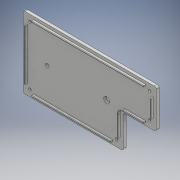
# Autodesk Inventor part: LID Enclosure Box
Saved by Autodesk Inventor 2017 (Build 210142000, 142)
## iProperties
Created: 2019-08-08
Part Number: LID Enclosure Box
Material: Generic
Document SubType Name: Modeling
Designer: harneet
Density: 1 g/cm^3
Appearance: Default
Author: harneet
Autodesk Inventor part; units mm, degrees
ref_plane "YZ Plane" through (0, 0, 0) normal (1, 0, 0) x (0, 1, 0)
ref_plane "XZ Plane" through (0, 0, 0) normal (0, 1, 0) x (-1, 0, 0)
ref_plane "XY Plane" through (0, 0, 0) normal (0, 0, 1) x (1, 0, 0)
sketch "Sketch1" plane through (0, 0, 0) normal (0, 1, 0) x (-1, 0, 0)
  line L0 (70.5, -36) -> (70.5, 36)
  line L1 (70.5, -38) -> (142.5, -38) construction
  line L2 (68.5, 38) -> (-68.5, 38)
  line L3 (-70.5, 36) -> (-70.5, -1)
  line L4 (-68.5, -3) -> (-37.5, -3)
  line L5 (68.5, -38) -> (-33.5, -38)
  line L6 (-35.5, -36) -> (-35.5, -5)
  arc A0 (70.5, 36) -> (68.5, 38) centre (68.5, 36) ccw
  arc A1 (68.5, -38) -> (70.5, -36) centre (68.5, -36) ccw
  arc A2 (-35.5, -36) -> (-33.5, -38) centre (-33.5, -36) ccw
  arc A3 (-35.5, -5) -> (-37.5, -3) centre (-37.5, -5) ccw
  arc A4 (-70.5, -1) -> (-68.5, -3) centre (-68.5, -1) ccw
  arc A5 (-68.5, 38) -> (-70.5, 36) centre (-68.5, 36) ccw
  point P0 (0, 0)
  point P1 (70.5, 38)
  point P2 (-70.5, 38)
  point P3 (-70.5, -3)
  point P4 (-35.5, -3)
  point P5 (-35.5, -38)
  dimension "d0" = 76
  dimension "d1" = 90
  dimension "d2" = 141
  dimension "d3" = 90
  dimension "d4" = 41
  dimension "d5" = 35
  dimension "d6" = 106
  dimension "d7" = 38
  dimension "d8" = 70.5
  dimension "d9" = 2
  constraints: 14 end point, 12 point on circle, 12 point on line, 12 tangent, 6 centre point, 5 equal radius, 4 perpendicular, 1 horizontal, 1 parallel, 1 vertical
  measures "d0" distance of L1.start point (70.5, 38)
  measures "d1" angle of L1 L0
  measures "d2" distance of point (70.5, 38) point (-70.5, 38)
  measures "d3" angle of L2 L0
  measures "d4" distance of point (-70.5, 38) point (-70.5, -3)
  measures "d5" distance of point (-70.5, -3) point (-35.5, -3)
  measures "d6" distance of L1.start point (-35.5, -38)
  measures "d7" distance from line of L5 point (0, 0)
  measures "d8" distance from line of L0 point (0, 0)
  measures "d9" radius of A0
extrude "Extrusion1" add sketch "Sketch1" along normal blind 3
sketch "Sketch2" plane through (0, 3, 0) normal (0, 1, 0) x (1, 0, 0)
  line L0 (-70.5, 36) -> (-70.5, -36) projected
  arc A0 (-70.5, -36) -> (-68.5, -38) centre (-68.5, -36) ccw projected
  line L1 (-68.5, -38) -> (68.5, -38) projected
  arc A1 (68.5, -38) -> (70.5, -36) centre (68.5, -36) ccw projected
  line L2 (70.5, -36) -> (70.5, 1) projected
  arc A2 (70.5, 1) -> (68.5, 3) centre (68.5, 1) ccw projected
  line L3 (68.5, 3) -> (37.5, 3) projected
  arc A3 (35.5, 5) -> (37.5, 3) centre (37.5, 5) ccw projected
  line L4 (35.5, 5) -> (35.5, 36) projected
  arc A4 (35.5, 36) -> (33.5, 38) centre (33.5, 36) ccw projected
  line L5 (33.5, 38) -> (-68.5, 38) projected
  arc A5 (-68.5, 38) -> (-70.5, 36) centre (-68.5, 36) ccw projected
  line L6 (-67.4, -27) -> (-67.4, 27)
  line L7 (-59.5, 34.9) -> (24.5, 34.9)
  line L8 (32.4, 27) -> (32.4, 5)
  arc A6 (32.4, 5) -> (37.5, -0.1) centre (37.5, 5) ccw
  line L9 (37.5, -0.1) -> (59.5, -0.1)
  line L10 (59.5, -34.9) -> (-59.5, -34.9)
  line L11 (0, 53.7799) -> (0, -53.7799) projected
  line L12 (99.2799, 0) -> (-99.2799, 0) projected
  line L13 (59.5, -33.5) -> (-59.5, -33.5)
  line L14 (-66, -27) -> (-66, 27)
  line L15 (-59.5, 33.5) -> (24.5, 33.5)
  line L16 (31, 27) -> (31, 5)
  arc A7 (31, 5) -> (37.5, -1.5) centre (37.5, 5) ccw
  line L17 (37.5, -1.5) -> (59.5, -1.5)
  line L18 (66, -8) -> (66, -27)
  line L19 (67.4, -8) -> (67.4, -27)
  line L20 (24.5, 34.9) -> (24.5, 33.5)
  line L21 (31, 27) -> (32.4, 27)
  line L22 (59.5, -1.5) -> (59.5, -0.1)
  line L23 (66, -8) -> (67.4, -8)
  line L24 (67.4, -27) -> (66, -27)
  line L25 (59.5, -33.5) -> (59.5, -34.9)
  line L26 (-59.5, -33.5) -> (-59.5, -34.9)
  line L27 (-67.4, -27) -> (-66, -27)
  line L28 (-66, 27) -> (-67.4, 27)
  line L29 (-59.5, 34.9) -> (-59.5, 33.5)
  point P0 (0, 0)
  dimension "d12" = 3.1
  dimension "d19" = 4.5
  dimension "d23" = 1.4
  dimension "d25" = 3.1
  dimension "d26" = 3.1
  dimension "d27" = 3.1
  dimension "d28" = 3.1
  dimension "d29" = 3.1
  dimension "d30" = 5.1
  dimension "d31" = 1.4
  dimension "d32" = 1.4
  dimension "d33" = 1.4
  dimension "d36" = 6.5
  dimension "d37" = 1.4
  constraints: 44 end point, 6 perpendicular, 4 point on circle, 3 parallel, 2 centre point, 1 vertical
  measures "d12" distance between parallel lines of L0 L6
  measures "d19" distance between parallel lines of L1 L13
  measures "d23" distance between parallel lines of L6 L14
  measures "d25" distance between parallel lines of L10 L1
  measures "d26" distance between parallel lines of L19 L2
  measures "d27" distance between parallel lines of L9 L3
  measures "d28" distance between parallel lines of L8 L4
  measures "d29" distance between parallel lines of L7 L5
  measures "d30" radius of A6
  measures "d31" distance between parallel lines of L9 L17
  measures "d32" distance between parallel lines of L19 L18
  measures "d33" distance between parallel lines of L7 L15
  measures "d36" radius of A7
  measures "d37" distance between parallel lines of L8 L16
extrude "Extrusion2" add sketch "Sketch2" along normal blind 2.5 contours L12 L14 L27 L6 | L6 L28 L14 L12 | L11 L15 L29 L7 | L7 L20 L15 L11 | L11 L13 L25 L10 | L10 L26 L13 L11 | A7 L16 L21 L8 A6 L12 | L12 A6 L9 L22 L17 A7 | L23 L19 L24 L18
fillet "Fillet1" radius 0.5 24 edges at (-67.4, 5.5, 0) (-66.7, 5.5, 27) (-66, 5.5, 0) (-66.7, 5.5, -27) (0, 5.5, 33.5) (-59.5, 5.5, 34.2) (0, 5.5, 34.9) (59.5, 5.5, 34.2) (-17.5, 5.5, -34.9) (-59.5, 5.5, -34.2) (-17.5, 5.5, -33.5) (24.5, 5.5, -34.2) (32.4, 5.5, -16) (31.7, 5.5, -27) (31, 5.5, -16) (32.9038, 5.5, -0.4038) (48.5, 5.5, 1.5) (59.5, 5.5, 0.8) (48.5, 5.5, 0.1) (33.8938, 5.5, -1.3938) (67.4, 5.5, 17.5) (66.7, 5.5, 8) (66, 5.5, 17.5) (66.7, 5.5, 27)
sketch "Sketch3" plane through (0, 3, 0) normal (0, 1, 0) x (1, 0, 0)
  circle A0 centre (-63.5, 31) radius 1.5
  circle A1 centre (-63.5, -31) radius 1.5
  circle A2 centre (63.5, -31) radius 1.5
  circle A3 centre (63.5, -4) radius 1.5
  circle A4 centre (28.5, 31) radius 1.5
  line L0 (33.5, 38) -> (-68.5, 38) projected
  line L1 (-70.5, 36) -> (-70.5, -36) projected
  line L2 (68.5, -38) -> (-68.5, -38) projected
  line L3 (35.5, 5) -> (35.5, 36) projected
  line L4 (68.5, 3) -> (37.5, 3) projected
  line L5 (70.5, -36) -> (70.5, 1) projected
  point P0 (0, 0)
  dimension "d41" = 3
  dimension "d42" = 3
  dimension "d43" = 3
  dimension "d44" = 3
  dimension "d45" = 3
  dimension "d46" = 7
  dimension "d47" = 7
  dimension "d48" = 7
  dimension "d49" = 7
  dimension "d50" = 7
  dimension "d51" = 7
  dimension "d52" = 7
  dimension "d53" = 7
  dimension "d54" = 7
  dimension "d55" = 7
  constraints: 5 centre point
  measures "d41" diameter of A0
  measures "d42" diameter of A1
  measures "d43" diameter of A2
  measures "d44" diameter of A3
  measures "d45" diameter of A4
  measures "d46" distance from line of L0 A0.centre
  measures "d47" distance from line of A0.centre L1
  measures "d48" distance from line of L2 A1.centre
  measures "d49" distance from line of L1 A1.centre
  measures "d50" distance from line of L0 A4.centre
  measures "d51" distance from line of A4.centre L3
  measures "d52" distance from line of A3.centre L4
  measures "d53" distance from line of A3.centre L5
  measures "d54" distance from line of L2 A2.centre
  measures "d55" distance from line of A2.centre L5
extrude "Extrusion3" cut sketch "Sketch3" against normal through all
chamfer "Chamfer2" distance 1.5 angle 45 5 edges at (-65, 3, 31) (-65, 3, -31) (27, 3, -31) (62, 3, 4) (62, 3, 31)
ref_plane "Work Plane3" through (0, 1.5, 0) normal (0, 1, 0) x (1, 0, 0)
mirror "Mirror1" about plane through (0, 1.5, 0) normal (0, 1, 0) of "Fillet1", "Extrusion2"
sketch "Sketch4" plane through (0, 3, 0) normal (0, 1, 0) x (1, 0, 0)
  circle A0 centre (18, 0) radius 3.185
  circle A1 centre (-45, 0) radius 2
  point P0 (0, 0)
  dimension "d65" = 6.37
  dimension "d66" = 4
  constraints: 2 centre point
  measures "d65" diameter of A0
  measures "d66" diameter of A1
extrude "Extrusion4" cut sketch "Sketch4" against normal blind 10
sketch "Sketch5" plane through (33.5, 0, -38) normal (0, 0, -1) x (-1, 0, 0)
  line L0 (-37, 0) -> (-37, 3) projected
  line L1 (-35, 3) -> (-4, 3) projected
  line L2 (104, 0) -> (104, 3) projected
  line L3 (-37, 3) -> (104, 3)
  line L4 (104, 3) -> (104, 8)
  line L5 (104, 8) -> (-37, 8)
  line L6 (-37, 8) -> (-37, 3)
  point P0 (33.5, 0)
  constraints: 8 end point, 2 parallel, 1 horizontal, 1 perpendicular
extrude "Extrusion5" cut sketch "Sketch5" against normal through all
equation "\"d7\" = 0.5 * d0"
equation "\"d8\" = 0.5 * d2"
equation "\"d23\" = d37"
equation "\"d31\" = d32"
equation "\"d33\" = d37"
body "Solid1"
